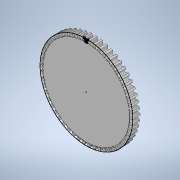
# Autodesk Inventor part: GearBig54T
Saved by Autodesk Inventor 2022 (Build 260153070, 153G)
## iProperties
Created: 2021-11-03
Part Number: GearBig54T
Material: Generic
Document SubType Name: Modeling
Designer: a laptop
Density: 1 g/cm^3
Appearance: Default
Author: a laptop
Autodesk Inventor part; units mm, degrees
ref_plane "YZ Plane" through (0, 0, 0) normal (1, 0, 0) x (0, 1, 0)
ref_plane "XZ Plane" through (0, 0, 0) normal (0, 1, 0) x (-1, 0, 0)
ref_plane "XY Plane" through (0, 0, 0) normal (0, 0, 1) x (1, 0, 0)
sketch "Sketch1" plane through (0, 0, 0) normal (0, 0, 1) x (1, 0, 0)
  spline S0 degree 3 poles (-0.763, 18.6095) (-0.7354, 18.5466) (-0.6801, 18.4208) (-0.6042, 18.229) (-0.5373, 18.0339) (-0.4458, 17.7757) (-0.4446, 17.5378) (-0.346, 17.395) (-0.3052, 17.3628) (-0.2577, 17.3412) (-0.1545, 17.3298) (0, 17.3425) (0.1545, 17.3298) (0.2577, 17.3412) (0.3052, 17.3628) (0.346, 17.395) (0.4446, 17.5378) (0.4458, 17.7757) (0.5373, 18.0339) (0.6042, 18.229) (0.6801, 18.4208) (0.7354, 18.5466) (0.763, 18.6095) knots 0 0 0 0 0.020613 0.041227 0.06184 0.082453 0.123616 0.12876 0.133903 0.139047 0.144189 0.164803 0.185417 0.190559 0.195703 0.200846 0.20599 0.247153 0.267766 0.288379 0.308992 0.329606 0.329606 0.329606 0.329606
  circle A0 centre (0, 0) radius 17.3368 construction
  circle A1 centre (0, 0) radius 17.2834 construction
  circle A2 centre (0, 0) radius 17.55 construction
  circle A3 centre (0, 0) radius 18.6251
  point P0 (-0.6812, 18.4203)
  point P1 (-0.6057, 18.2285)
  point P2 (-0.537, 18.0341)
  point P3 (-0.4761, 17.8372)
  point P4 (-0.3745, 17.4383)
  point P5 (-0.3441, 17.3968)
  point P6 (-0.3041, 17.3645)
  point P7 (-0.257, 17.3438)
  point P8 (-0.2061, 17.3361)
  point P9 (0, 17.3368)
  point P10 (0.2061, 17.3361)
  point P11 (0.257, 17.3438)
  point P12 (0.3041, 17.3645)
  point P13 (0.3441, 17.3968)
  point P14 (0.3745, 17.4383)
  point P15 (0.4761, 17.8372)
  point P16 (0.537, 18.0341)
  point P17 (0.6057, 18.2285)
  point P18 (0.6812, 18.4203)
  constraints: 4 centre point, 2 point on circle, 47 other
extrude "Extrusion1" add sketch "Sketch1" against normal blind 3
extrude "Extrusion2" cut sketch "Sketch1" against normal blind 10 contours A3 S0 picked at (0.0921, 18.2082)
pattern_circular "Circular Pattern1" count 54 over 360 about axis through (0, 0, 0) along (0, 0, -1) of "Extrusion2"
equation "\"d0\" = FaceWidth"
equation "\"Module\" = 0.65"
equation "\"PressureAngle\" = 10deg"
equation "\"UnitProfileClearance\" = 0.25"
equation "\"UnitRoundRadius\" = 0.3025"
equation "\"HeadDiameter\" = 37.25022"
equation "\"RootDiameter\" = 34.67367"
equation "\"BaseDiameter\" = 34.56675"
equation "\"PitchDiameter\" = 35.1"
equation "\"FaceWidth\" = 3"
equation "\"HelixAngle\" = 0"
equation "\"UnitCorrection\" = 0.922054"
equation "\"UnitAddendumModification\" = 0.268038"
equation "\"CircularPitch\" = 2.04204"
equation "\"UnitBacklashShift\" = 0"
equation "\"TotalToolShift\" = 0.59934"
equation "\"IsInternal\" = 0"
body "Solid1"
